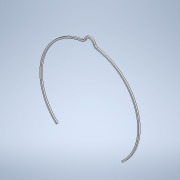
# Autodesk Inventor part: 69. Пружина синхронизатора
Saved by Autodesk Inventor 2021 (Build 250183000, 183)
## iProperties
Created: 2021-03-22
Part Number: 69. Пружина синхронизатора
Material: Типовые
Document SubType Name: Modeling
Designer: Данил
Density: 1 g/cm^3
Appearance: По умолчанию
Author: Данил
Autodesk Inventor part; units mm, degrees
ref_plane "YZ Plane" through (0, 0, 0) normal (1, 0, 0) x (0, 1, 0)
ref_plane "XZ Plane" through (0, 0, 0) normal (0, 1, 0) x (-1, 0, 0)
ref_plane "XY Plane" through (0, 0, 0) normal (0, 0, 1) x (1, 0, 0)
sketch "Эскиз1" plane through (0, 0, 0) normal (0, 0, 1) x (1, 0, 0)
  circle A0 centre (0, 0) radius 37
  circle A1 centre (0, 0) radius 36
  arc A2 (-5.4946, 36.5897) -> (-3.8611, 38.045) centre (-5.7916, 38.5676) ccw
  arc A3 (3.8611, 38.045) -> (-3.8611, 38.045) centre (0, 37) ccw
  arc A4 (3.8611, 38.045) -> (5.4946, 36.5897) centre (5.7916, 38.5676) ccw
  line L0 (-24, -26.8328) -> (24, -26.8328) construction
  line L1 (-24, -26.8328) -> (-24.7499, -27.5035)
  line L2 (24, -26.8328) -> (24.6667, -27.5782)
  arc A5 (-5.3461, 35.6008) -> (-2.8958, 37.7838) centre (-5.7916, 38.5676) ccw
  arc A6 (2.8958, 37.7838) -> (-2.8958, 37.7838) centre (0, 37) ccw
  arc A7 (2.8958, 37.7838) -> (5.3461, 35.6008) centre (5.7916, 38.5676) ccw
  point P0 (5.3461, 35.6008)
  dimension "d0" = 74
  dimension "d1" = 72
  dimension "d2" = 4
  dimension "d4" = 2
  dimension "d5" = 48
  constraints: 19 point on circle, 8 centre point, 6 end point, 5 tangent, 2 coincident, 1 equal radius, 1 horizontal, 1 horizontal alignment, 1 line through centre, 1 perpendicular, 2 other
  measures "d0" diameter of A0
  measures "d1" diameter of A1
  measures "d2" radius of A3
  measures "d4" radius of A4
  measures "d5" distance of L0.start L0.end
extrude "Выдавливание1" add sketch "Эскиз1" along normal mid plane 1 contours A0 L2 A1 A7 | A0 A7 A6 A5 A2 A3 A4 | A0 A5 A1 L1
